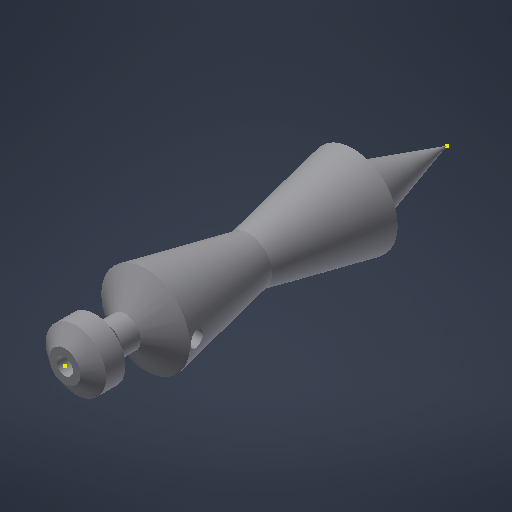
# Autodesk Inventor part: BAILARINA
Saved by Autodesk Inventor 2026 (Build 300175000, 175)
## iProperties
Created: 2025-03-28
Part Number: BAILARINA
Material: Generic
Document SubType Name: Modeling
Designer: usuario
Density: 1 g/cm^3
Appearance: Default
Author: usuario
Autodesk Inventor part; units mm, degrees
ref_plane "YZ Plane" through (0, 0, 0) normal (1, 0, 0) x (0, 1, 0)
ref_plane "XZ Plane" through (0, 0, 0) normal (0, 1, 0) x (-1, 0, 0)
sketch "Boceto1" plane through (0, 0, 0) normal (1, 0, 0) x (0, 1, 0)
  point P0 (0, 0)
sketch "Boceto2" plane through (0, 0, 0) normal (1, 0, 0) x (0, 1, 0)
  point P0 (0, 0)
  point P1 (0, 0)
  constraints: 1 coincident
ref_plane "Plano de trabajo1" through (0, 0, 19.45) normal (0, 0, 1) x (1, 0, 0)
sketch "Boceto3" plane through (0, 0, 19.45) normal (0, 0, 1) x (1, 0, 0)
  circle A0 centre (0, 0) radius 5.825
  dimension "d1" = 11.65
  constraints: 1 centre point, 1 coincident
  measures "d1" diameter of A0
ref_plane "Plano de trabajo3" through (0, 0, 62.35) normal (0, 0, 1) x (1, 0, 0)
ref_plane "Plano de trabajo2" through (0, 0, 41) normal (0, 0, 1) x (1, 0, 0)
sketch "Boceto4" plane through (0, 0, 19.45) normal (0, 0, 1) x (1, 0, 0)
  circle A0 centre (0, 0) radius 9.225
  dimension "d4" = 18.45
  constraints: 1 centre point, 1 coincident
  measures "d4" diameter of A0
sketch "Boceto5" plane through (0, 0, 41) normal (0, 0, 1) x (1, 0, 0)
  circle A0 centre (0, 0) radius 4.8
  dimension "d5" = 9.6
  constraints: 1 centre point, 1 coincident
  measures "d5" diameter of A0
sketch "Boceto6" plane through (0, 0, 62.35) normal (0, 0, 1) x (1, 0, 0)
  circle A0 centre (0, 0) radius 9.175
  dimension "d6" = 18.35
  constraints: 1 centre point, 1 coincident
  measures "d6" diameter of A0
ref_plane "Plano de trabajo4" through (0, 0, 66.55) normal (0, 0, 1) x (1, 0, 0)
sketch "Boceto7" plane through (0, 0, 66.55) normal (0, 0, 1) x (1, 0, 0)
  point P0 (0, 0)
sketch "Boceto8" plane through (0, 0, 66.55) normal (0, 0, 1) x (1, 0, 0)
  circle A0 centre (0, 0) radius 3.225
  dimension "d8" = 6.45
  constraints: 1 centre point, 1 coincident
  measures "d8" diameter of A0
ref_plane "Plano de trabajo5" through (0, 0, 70.4) normal (0, 0, 1) x (1, 0, 0)
sketch "Boceto9" plane through (0, 0, 70.4) normal (0, 0, 1) x (1, 0, 0)
  circle A0 centre (0, 0) radius 3.225
  dimension "d10" = 6.45
  constraints: 1 centre point, 1 coincident
  measures "d10" diameter of A0
loft "Solevación1" add profiles "Boceto3" section 1 point at (0, 0, 0)
loft "Solevación2" add profiles "Boceto4", "Boceto5"
loft "Solevación3" add profiles "Boceto6" section 1 edges at (-4.8, 0, 41)
loft "Solevación4" add profiles "Boceto8" section 1 edges at (-9.175, 0, 62.35)
loft "Solevación5" add profiles "Boceto9" section 1 edges at (-3.225, 0, 66.55)
ref_plane "Plano de trabajo8" through (0, 0, 79.05) normal (0, 0, 1) x (1, 0, 0)
ref_plane "Plano de trabajo7" through (0, 0, 76.75) normal (0, 0, 1) x (1, 0, 0)
sketch "Boceto10" plane through (0, 0, 72.75) normal (0, 0, 1) x (1, 0, 0)
  circle A0 centre (0, 0) radius 6.25
  dimension "d34" = 12.5
  constraints: 1 centre point, 1 coincident
  measures "d34" diameter of A0
sketch "Boceto11" plane through (0, 0, 76.75) normal (0, 0, 1) x (1, 0, 0)
  circle A0 centre (0, 0) radius 6.25
  dimension "d35" = 12.5
  constraints: 1 centre point, 1 coincident
  measures "d35" diameter of A0
sketch "Boceto12" plane through (0, 0, 79.05) normal (0, 0, 1) x (1, 0, 0)
  point P0 (0, 0)
sketch "Boceto13" plane through (0, 0, 79.05) normal (0, 0, 1) x (1, 0, 0)
  circle A0 centre (0, 0) radius 3.225
  dimension "d36" = 6.45
  constraints: 1 centre point, 1 coincident
  measures "d36" diameter of A0
loft "Solevación6" add profiles "Boceto10" section 1 edges at (-3.225, 0, 70.4)
loft "Solevación7" add profiles "Boceto11" section 1 edges at (-6.25, 0, 72.75)
loft "Solevación8" add profiles "Boceto13" section 1 edges at (-6.25, 0, 76.75)
sketch "Boceto14" plane through (0, 0, 79.05) normal (0, 0, 1) x (1, 0, 0)
  circle A0 centre (0, 0) radius 1.7
  dimension "d49" = 3.4
  constraints: 1 centre point, 1 coincident
  measures "d49" diameter of A0
extrude "Extrusión1" cut sketch "Boceto14" against normal blind 2.75
sketch "Sketch15" plane through (0, 0, 0) normal (1, 0, 0) x (0, 1, 0)
  circle A0 centre (0, 60.5) radius 1.59
  point P0 (0, 0)
  dimension "d52" = 3.18
  dimension "d53" = 60.5
  constraints: 1 centre point, 1 vertical alignment
  measures "d52" diameter of A0
  measures "d53" distance of point (0, 0) A0.centre
extrude "Extrusion2" cut sketch "Sketch15" along normal through all both and the other way through all
ref_plane "Plano de trabajo6" through (0, 0, 72.75) normal (0, 0, 1) x (1, 0, 0)
